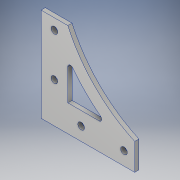
# Autodesk Inventor part: Corner Bracket
Saved by Autodesk Inventor 2019.1 (Build 231200000, 200)
## iProperties
Created: 2018-08-19
Part Number: Corner Bracket
Material: Aluminum 6061
Document SubType Name: Modeling
Designer: Richard
Density: 2.7 g/cm^3
Appearance: Aluminum - Flat
Author: Richard
Autodesk Inventor part; units mm, degrees
ref_plane "YZ Plane" through (0, 0, 0) normal (1, 0, 0) x (0, 1, 0)
ref_plane "XZ Plane" through (0, 0, 0) normal (0, 1, 0) x (-1, 0, 0)
ref_plane "XY Plane" through (0, 0, 0) normal (0, 0, 1) x (1, 0, 0)
sketch "Sketch1" plane through (0, 0, 0) normal (0, 0, 1) x (1, 0, 0)
  line L0 (0, 0) -> (0, 70)
  line L1 (0, 70) -> (20, 70)
  line L2 (0, 0) -> (70, 0)
  line L3 (70, 0) -> (70, 20)
  arc A0 (20, 70) -> (70, 20) centre (111.1438, 111.1438) ccw
  arc A1 (23.5919, 44.5505) -> (44.5505, 23.5919) centre (111.1438, 111.1438) ccw
  line L4 (20, 43.3398) -> (20, 20)
  line L5 (20, 20) -> (43.3398, 20)
  arc A2 (23.5919, 44.5505) -> (20, 43.3398) centre (22, 43.3398) ccw
  arc A3 (43.3398, 20) -> (44.5505, 23.5919) centre (43.3398, 22) ccw
  line L6 (10, 62) -> (10, 30) construction
  line L7 (62, 10) -> (30, 10) construction
  circle A4 centre (10, 62) radius 2.5
  circle A5 centre (10, 30) radius 2.5
  circle A6 centre (30, 10) radius 2.5
  circle A7 centre (62, 10) radius 2.5
  point P0 (70, 10)
  point P1 (10, 70)
  dimension "d0" = 70
  dimension "d1" = 70
  dimension "d2" = 20
  dimension "d4" = 100
  dimension "d5" = 10
  dimension "d6" = 2
  dimension "d7" = 32
  dimension "d8" = 32
  dimension "d9" = 8
  dimension "d10" = 8
  dimension "d11" = 5
  dimension "d12" = 5
  dimension "d13" = 5
  dimension "d14" = 5
  constraints: 16 end point, 8 centre point, 8 point on circle, 4 coincident, 4 perpendicular, 4 point on line, 4 tangent, 3 vertical, 2 horizontal, 2 midpoint, 1 concentric, 1 equal radius
  measures "d0" distance of L0.start L0.end
  measures "d1" distance of L0.start L2.end
  measures "d2" distance of L0.end L1.end
  measures "d4" radius of A0
  measures "d5" radial gap between concentric circles of A0 A1
  measures "d6" radius of A2
  measures "d7" distance of L6.start L6.end
  measures "d8" distance of L7.start L7.end
  measures "d9" distance from line of L1 L6.start
  measures "d10" distance from line of L3 L7.start
  measures "d11" diameter of A4
  measures "d12" diameter of A5
  measures "d13" diameter of A6
  measures "d14" diameter of A7
extrude "Extrusion1" add sketch "Sketch1" along normal mid plane 3.175
equation "\"d10\" = d9"
body "Solid1"
